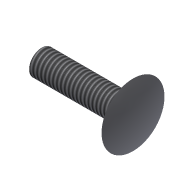
# Autodesk Inventor part: Šroub M8x24
Saved by Autodesk Inventor 2015 (Build 190159000, 159)
## iProperties
Created: 2015-01-15
Part Number: Šroub M8x24
Material: Všeobecné
Document SubType Name: Modeling
Designer: Michal
Density: 1 g/cm^3
Appearance: Výchozí
Author: Michal
Autodesk Inventor part; units mm, degrees
ref_plane "YZ Plane" through (0, 0, 0) normal (1, 0, 0) x (0, 1, 0)
ref_plane "XZ Plane" through (0, 0, 0) normal (0, 1, 0) x (-1, 0, 0)
ref_plane "XY Plane" through (0, 0, 0) normal (0, 0, 1) x (1, 0, 0)
sketch "Náčrt1" plane through (0, 0, 0) normal (1, 0, 0) x (0, 1, 0)
  circle A0 centre (0, 0) radius 4
  dimension "d0" = 8
  constraints: 1 centre point, 1 coincident
  measures "d0" diameter of A0
extrude "Vysunutí1" add sketch "Náčrt1" along normal blind 29
sketch "Náčrt2" plane through (0, 0, 0) normal (0, 1, 0) x (-1, 0, 0)
  line L0 (-29, 4) -> (-29, -4) projected
  line L1 (0, -4) -> (0, 4) projected
  line L2 (-29, 0) -> (-29, -10)
  arc A0 (-30.6757, 0) -> (-29, -10) centre (0, 0) ccw
  line L3 (-29, 0) -> (-30.6757, 0)
  dimension "d3" = 10
  constraints: 4 end point, 2 point on circle, 1 centre point, 1 coincident, 1 midpoint, 1 vertical
  measures "d3" distance of L2.start L2.end
revolve "Rotace1" add sketch "Náčrt2" angle 360 about axis through (29, 0, 0) along (1, 0, 0)
thread "Závit1" size "M8x1.25" class "6g" standard "ANSI Metric M Profile" full length
